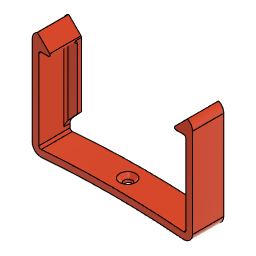
mounting_bracket (Autodesk Fusion 360 design; units mm, degrees)
Autodesk Fusion 360 part; units mm, degrees
sketch "Sketch1" plane through (0, 0, 0) normal (0, 1, 0) x (1, 0, 0) in component "Base Model"
  line L0 (-35, -40) -> (35, -40) construction
  line L1 (35, -40) -> (35, 0) construction
  line L2 (35, 0) -> (-35, 0) construction
  line L3 (-35, 0) -> (-35, -40) construction
  line L4 (35.3, -40.3) -> (-35.3, -40.3)
  line L5 (-35.3, -40.3) -> (-35.3, 0.3)
  line L6 (-35.3, 0.3) -> (35.3, 0.3) construction
  line L7 (35.3, 0.3) -> (35.3, -40.3)
  line L8 (-38.5, -50.1) -> (-28.7, -40.3)
  arc A0 (-35.3, 0.3) -> (35.3, 0.3) centre (0, 403.7808) ccw
  line L9 (0, -40) -> (0, 0)
  line L10 (-35.3, 0.3) -> (0, -2.7883) construction
  line L11 (-38.5, -40.3) -> (-38.5, 3.8074)
  arc A1 (-38.5, 3.8074) -> (38.5, 3.8074) centre (0, 403.7808) ccw
  line L12 (38.5, 3.8074) -> (38.5, -40.3)
  line L13 (-38.5, -50.1) -> (-38.5, -40.3)
  line L14 (-36, -47.6) -> (-38.5, -47.6)
  line L15 (38.5, -50.1) -> (38.5, -40.3)
  line L16 (36, -47.6) -> (38.5, -47.6)
  line L17 (38.5, -50.1) -> (28.7, -40.3)
  dimension "d1" = 40
  dimension "d2" = 70
  dimension "d4" = 0.3
  dimension "d11" = 0.3
  dimension "d12" = 0.3
  dimension "d18" = 0.3
  dimension "d40" = 45
  dimension "d44" = 85
  dimension "d52" = 6.6
  dimension "d57" = 1
  constraint horizontal L0
  constraint horizontal L2
  constraint vertical L3
  constraint midpoint L9.end L2
  constraint horizontal L6
  constraint vertical L5
  constraint horizontal L4
  constraint perpendicular L6 L7
  constraint midpoint L0 L9.start
  constraint coincident L9.end origin
  constraint coincident L9 L10.end
  constraint tangent A0 L10
  constraint coincident L4.start L7.end
  constraint coincident L4 L8.end
  constraint vertical L13
  constraint coincident L8.start L13.start
  constraint coincident L8 L14.start
  constraint coincident L13 L14.end
  constraint perpendicular L13 L14
  constraint symmetric L8.start L9 L15.start
  constraint symmetric L8.end L9 L17.end
  constraint symmetric L9 L11.start L12.end
  constraint symmetric L9 L14.start L16.start
  constraint symmetric L9 L14.end L16.end
  measures "d1" distance of L0 L2
  measures "d2" distance of L1 L3
  measures "d4" distance of L3 L5
  measures "d11" distance of L2 L6
  measures "d12" distance of L1 L6.end
  measures "d18" distance of L0 L4
  measures "d40" angle of L4 L8
  measures "d44" angle of L5 L10
  measures "d52" distance of L5 L8.end
  measures "d57" distance of L3 L14.start
extrude "Extrude1" add sketch "Sketch1" along normal blind 15 contours L4 L5 L7 L8 A0 L11 A1 L12 L13 L14 L15 L16 L17 makes body 1 in component "Base Model"
fillet "Fillet1" radius 1 4 edges at (35.3, 7.5, -0.3) (-35.3, 7.5, 40.3) (-35.3, 7.5, -0.3) (35.3, 7.5, 40.3) on bodies 1 in component "Base Model"
fillet "Fillet2" radius 4.2 4 edges at (-38.5, 7.5, -3.8074) (38.5, 7.5, -3.8074) (-38.5, 7.5, 47.6) (38.5, 7.5, 47.6) on bodies 1 in component "Base Model"
fillet "Fillet3" radius 0.8 2 edges at (-28.7, 7.5, 40.3) (28.7, 7.5, 40.3) on bodies 1 in component "Base Model"
ref_plane "WorkPlane1" through (-12.4016, 3.6685, 1.0513) normal (-0.03062, 0, 0.999531) x (-0.999531, 0, -0.03062) in component "Base Model"
sketch "Sketch2" plane through (-12.4016, 3.6685, 1.0513) normal (-0.03062, 0, 0.999531) x (0.999531, 0, 0.03062) in component "Base Model"
  line L0 (-21.8422, 11.3315) -> (-21.8422, -3.6685)
  line L1 (46.5568, -3.6685) -> (-21.8422, -3.6685)
  line L2 (46.5568, -3.6685) -> (46.5568, 11.3315)
  line L3 (46.5568, 11.3315) -> (-21.8422, 11.3315)
  line L4 (46.5568, -3.6685) -> (-21.8422, 11.3315) construction
  circle A0 centre (12.3573, 3.8315) radius 2.15
  dimension "d29" = 4.3
  constraint coincident L1.start L2.start
  constraint coincident L0.start L3.end
  constraint midpoint L4 A0.centre
  measures "d29" diameter of A0
hole "Hole1" at (-0.0501, 7.5, 1.4297) direction (0.03062, 0, -0.999531) diameter 4 depth 7 tip angle 118 countersink diameter 8 countersink angle 90 bodies 1 in component "Base Model"
sketch "Sketch1 (2)" plane through (0, 0, 0) normal (0, 1, 0) x (1, 0, 0) in component "Vertical Model"
  line L0 (-35, -40) -> (35, -40) construction
  line L1 (35, -40) -> (35, 0) construction
  line L2 (35, 0) -> (-35, 0) construction
  line L3 (-35, 0) -> (-35, -40) construction
  line L4 (35.3, -40.3) -> (-35.3, -40.3)
  line L5 (-35.3, -40.3) -> (-35.3, 0.3)
  line L6 (-35.3, 0.3) -> (35.3, 0.3) construction
  line L7 (35.3, 0.3) -> (35.3, -40.3)
  line L8 (-38.5, -50.1) -> (-28.7, -40.3)
  arc A0 (-35.3, 0.3) -> (35.3, 0.3) centre (0, 403.7808) ccw
  line L9 (0, -40) -> (0, 0)
  line L10 (-35.3, 0.3) -> (0, -2.7883) construction
  line L11 (-38.5, -40.3) -> (-38.5, 3.8074)
  arc A1 (-38.5, 3.8074) -> (38.5, 3.8074) centre (0, 403.7808) ccw
  line L12 (38.5, 3.8074) -> (38.5, -40.3)
  line L13 (-38.5, -50.1) -> (-38.5, -40.3)
  line L14 (-36, -47.6) -> (-38.5, -47.6)
  line L15 (38.5, -50.1) -> (38.5, -40.3)
  line L16 (36, -47.6) -> (38.5, -47.6)
  line L17 (38.5, -50.1) -> (28.7, -40.3)
  dimension "d1_1" = 40
  dimension "d2_1" = 70
  dimension "d4_1" = 0.3
  dimension "d11_1" = 0.3
  dimension "d12_1" = 0.3
  dimension "d18_1" = 0.3
  dimension "d40_1" = 45
  dimension "d44_1" = 85
  dimension "d52_1" = 6.6
  dimension "d57_1" = 1
  constraint horizontal L0
  constraint horizontal L2
  constraint vertical L3
  constraint midpoint L9.end L2
  constraint horizontal L6
  constraint vertical L5
  constraint horizontal L4
  constraint perpendicular L6 L7
  constraint midpoint L0 L9.start
  constraint coincident L9.end origin
  constraint coincident L9 L10.end
  constraint tangent A0 L10
  constraint coincident L4.start L7.end
  constraint coincident L4 L8.end
  constraint vertical L13
  constraint coincident L8.start L13.start
  constraint coincident L8 L14.start
  constraint coincident L13 L14.end
  constraint perpendicular L13 L14
  constraint symmetric L8.start L9 L15.start
  constraint symmetric L8.end L9 L17.end
  constraint symmetric L9 L11.start L12.end
  constraint symmetric L9 L14.start L16.start
  constraint symmetric L9 L14.end L16.end
  measures "d1_1" distance of L0 L2
  measures "d2_1" distance of L1 L3
  measures "d4_1" distance of L3 L5
  measures "d11_1" distance of L2 L6
  measures "d12_1" distance of L1 L6.end
  measures "d18_1" distance of L0 L4
  measures "d40_1" angle of L4 L8
  measures "d44_1" angle of L5 L10
  measures "d52_1" distance of L5 L8.end
  measures "d57_1" distance of L3 L14.start
extrude "Extrude1'" add sketch "Sketch1 (2)" along normal blind 15 separate body contours L4 L5 L7 L8 A0 L11 A1 L12 L13 L14 L15 L16 L17 makes body 2 in component "Vertical Model"
fillet "Fillet1'" radius 1 4 edges at (35.3, 7.5, -0.3) (-35.3, 7.5, 40.3) (-35.3, 7.5, -0.3) (35.3, 7.5, 40.3) on bodies 2 in component "Vertical Model"
fillet "Fillet2'" radius 4.2 4 edges at (-38.5, 7.5, -3.8074) (38.5, 7.5, -3.8074) (-38.5, 7.5, 47.6) (38.5, 7.5, 47.6) on bodies 2 in component "Vertical Model"
fillet "Fillet3'" radius 0.8 2 edges at (-28.7, 7.5, 40.3) (28.7, 7.5, 40.3) on bodies 2 in component "Vertical Model"
ref_plane "WorkPlane1" through (-12.4016, 3.6685, 1.0513) normal (-0.03062, 0, 0.999531) x (-0.999531, 0, -0.03062) in component "Vertical Model"
sketch "Sketch2 (2)" plane through (-12.4016, 3.6685, 1.0513) normal (-0.03062, 0, 0.999531) x (0.999531, 0, 0.03062) in component "Vertical Model"
  line L0 (-21.8422, 11.3315) -> (-21.8422, -3.6685)
  line L1 (46.5568, -3.6685) -> (-21.8422, -3.6685)
  line L2 (46.5568, -3.6685) -> (46.5568, 11.3315)
  line L3 (46.5568, 11.3315) -> (-21.8422, 11.3315)
  line L4 (46.5568, -3.6685) -> (-21.8422, 11.3315) construction
  circle A0 centre (12.3573, 3.8315) radius 2.15
  dimension "d29_1" = 4.3
  constraint coincident L1.start L2.start
  constraint coincident L0.start L3.end
  constraint midpoint L4 A0.centre
  measures "d29_1" diameter of A0
hole "Hole1'" at (-0.0501, 7.5, 1.4297) direction (0.03062, 0, -0.999531) diameter 4 depth 7 tip angle 118 countersink diameter 8 countersink angle 90 bodies 2 in component "Vertical Model"
sketch "Sketch1 (1)" plane through (0, 15, 0) normal (0, 1, 0) x (-1, 0, 0) in component "Vertical Model"
  arc A0 (-30.6314, 40.3) -> (-30.0657, 41.6657) centre (-30.6314, 41.1) ccw
  line L0 (-30.0657, 41.6657) -> (-36, 47.6)
  arc A1 (-36, 47.6) -> (-38.5, 43.7594) centre (-34.3, 43.7594) ccw
  line L1 (-38.5, 43.7594) -> (-38.5, 0.7898)
  arc A2 (-38.5, 0.7898) -> (-33.9452, -3.3951) centre (-34.3, 0.7898) ccw
  arc A3 (33.9452, -3.3951) -> (-33.9452, -3.3951) centre (0, -403.7808) ccw
  arc A4 (33.9452, -3.3951) -> (38.5, 0.7898) centre (34.3, 0.7898) ccw
  line L2 (38.5, 0.7898) -> (38.5, 43.7594)
  arc A5 (38.5, 43.7594) -> (36, 47.6) centre (34.3, 43.7594) ccw
  line L3 (36, 47.6) -> (30.0657, 41.6657)
  arc A6 (30.0657, 41.6657) -> (30.6314, 40.3) centre (30.6314, 41.1) ccw
  line L4 (30.6314, 40.3) -> (34.3, 40.3)
  arc A7 (35.3, 39.3) -> (34.3, 40.3) centre (34.3, 39.3) ccw
  line L5 (35.3, 39.3) -> (35.3, 0.7898)
  arc A8 (34.2155, -0.2066) -> (35.3, 0.7898) centre (34.3, 0.7898) ccw
  arc A9 (34.2155, -0.2066) -> (-34.2155, -0.2066) centre (0, -403.7808) ccw
  arc A10 (-35.3, 0.7898) -> (-34.2155, -0.2066) centre (-34.3, 0.7898) ccw
  line L6 (-35.3, 0.7898) -> (-35.3, 39.3)
  arc A11 (-34.3, 40.3) -> (-35.3, 39.3) centre (-34.3, 39.3) ccw
  line L7 (-34.3, 40.3) -> (-30.6314, 40.3)
  line L8 (-37.1416, -2.3029) -> (-29.8314, 5.6534)
  line L9 (-29.8314, 5.6534) -> (-29.8314, 41.1)
  line L10 (-29.8314, 10.2245) -> (-38.5, 0.7898)
  constraint midpoint A2 L8.start
  constraint parallel L6 L9
  constraint symmetric A9.end A10.start L8
  constraint coincident L9 L10.start
  constraint parallel L8 L10
  constraint coincident L1.end A2.start
  constraint coincident A0 L9.end
  constraint tangent A0 L9
extrude "Extrude1''" add sketch "Sketch1 (1)" against normal blind 2 contours A0 L6 A11 L7 L9 L10 bodies 2 in component "Vertical Model"
ref_plane "WorkPlane1" through (0, 7.5, 22.2746) normal (1, 0, 0) x (0, 0, -1) in component "Vertical Model"
mirror "Mirror1" about plane through (0, 7.5, 22.2746) normal (1, 0, 0) of "Extrude1''" in component "Vertical Model"
fillet "Fillet1''" radius 1 8 edges at (30.0657, 13, 40.5343) (32.4657, 13, 40.3) (35.0071, 13, 40.0071) (35.3, 13, 21.7863) (-35.3, 13, 21.7863) (-35.0071, 13, 40.0071) (-32.4657, 13, 40.3) (-30.0657, 13, 40.5343) on bodies 2 in component "Vertical Model"
fillet "Fillet2''" radius 4.2 2 edges at (35.3, 13.5, 4.2726) (-35.3, 13.5, 4.2726) on bodies 2 in component "Vertical Model"
component "Base Model" placed x (1, 0, 0) y (0, 1, 0) z (0, 0, 1) at (0, 0, 0)
component "Vertical Model" placed x (1, 0, 0) y (0, 1, 0) z (0, 0, 1) at (0, 0, 0)
equation "d1 = height"
equation "d2 = width"
equation "d4 = clearance"
equation "d11 = clearance"
equation "d12 = clearance"
equation "d20 = -wallThickness"
equation "d25 = fillet"
equation "height = 40 mm" comment "Height of the device to hold"
equation "width = 70 mm" comment "Width of the device to hold"
equation "wallThickness = floor(targetWallThickness / ( 2 * nozzleWidth )) * 2 * nozzleWidth" comment "Enforces an even count of perimeters"
equation "overhang = 5 mm" comment "Overhang that wraps around the device"
equation "clearance = 0.3 mm" comment "Clearance between the bracket and the device"
equation "nozzleWidth = 0.8 mm"
equation "targetWallThickness = 3.5 mm"
equation "d44 = 90 deg - clampAngle / 2"
equation "clampAngle = 10 deg"
equation "fillet = 1 mm"
equation "d51 = -wallThickness"
equation "d52 = overhang + 2 * nozzleWidth"
equation "d54 = fillet + wallThickness"
equation "d56 = nozzleWidth"
equation "d1_1 = height"
equation "d2_1 = width"
equation "d4_1 = clearance"
equation "d11_1 = clearance"
equation "d12_1 = clearance"
equation "d25_1 = fillet"
equation "d44_1 = 90 deg - clampAngle / 2"
equation "d51_1 = -wallThickness"
equation "d52_1 = overhang + 2 * nozzleWidth"
equation "d54_1 = fillet + wallThickness"
equation "d56_1 = nozzleWidth"
equation "d71 = fillet"
equation "d75 = wallThickness + fillet"
